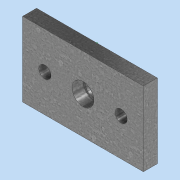
# Autodesk Inventor part: Unten
Saved by Autodesk Inventor 2021 (Build 250183000, 183)
## iProperties
Created: 2024-03-13
Part Number: Unten
Material: Generic
Document SubType Name: Modeling
Designer: Nokia
Density: 1 g/cm^3
Appearance: Steel Galvanized
Mass: 1145.79 g
Surface Area: 1212.7 cm^2
Volume: 1145.79 cm^3
Author: Nokia
Autodesk Inventor part; units mm, degrees
ref_plane "YZ Plane" through (0, 0, 0) normal (1, 0, 0) x (0, 1, 0)
ref_plane "XZ Plane" through (0, 0, 0) normal (0, 1, 0) x (-1, 0, 0)
ref_plane "XY Plane" through (0, 0, 0) normal (0, 0, 1) x (1, 0, 0)
sketch "Sketch1" plane through (0, 0, 0) normal (0, 0, 1) x (1, 0, 0)
  line L0 (130, -80) -> (130, 80)
  line L1 (130, 80) -> (-130, 80)
  line L2 (-130, 80) -> (-130, -80)
  line L3 (-130, -80) -> (130, -80)
  point P0 (0, 0)
  point P1 (0, 0)
  dimension "d0" = 260
  dimension "d1" = 160
  constraints: 8 end point, 3 perpendicular
  measures "d0" distance of L0.end L1.end
  measures "d1" distance of L1.end L2.end
extrude "Extrusion1" add sketch "Sketch1" along normal blind 30
sketch "Sketch2" plane through (0, 0, 30) normal (0, 0, 1) x (1, 0, 0)
  circle A0 centre (0, 0) radius 20
  circle A1 centre (0, 0) radius 23.5
  dimension "d4" = 40
  dimension "d5" = 47
  constraints: 2 centre point, 2 coincident
  measures "d4" diameter of A0
  measures "d5" diameter of A1
extrude "Extrusion2" cut sketch "Sketch2" against normal blind 30 contours A0
extrude "Extrusion3" cut sketch "Sketch2" against normal blind 24
sketch "Sketch3" plane through (0, 0, 30) normal (0, 0, 1) x (1, 0, 0)
  line L0 (-130, 80) -> (-130, -80) projected
  circle A0 centre (-82, 0) radius 13
  circle A1 centre (82, 0) radius 13
  line L1 (130, -80) -> (130, 80) projected
  point P0 (0, 0)
  dimension "d11" = 26
  dimension "d14" = 48
  dimension "d15" = 48
  constraints: 2 centre point
  measures "d11" diameter of A0
  measures "d14" distance from line of L0 A0.centre
  measures "d15" distance from line of L1 A1.centre
extrude "Extrusion4" cut sketch "Sketch3" against normal through all
sketch "Sketch4" plane through (-130, 80, 0) normal (0, 1, 0) x (1, 0, 0)
  point P0 (130, 0)
sketch "Sketch7" plane through (-130, -80, 0) normal (0, -1, 0) x (1, 0, 0)
  line L0 (260, 0) -> (0, 0)
  line L1 (0, 0) -> (0, 30)
  line L2 (130, 30) -> (260, 30)
  line L3 (130, 30) -> (130, 0)
  line L4 (195, 81.0719) -> (195, -34.56)
  line L5 (130, 15) -> (195, 15)
  line L6 (162.5, 115.0039) -> (162.5, -41.4165)
  circle A0 centre (162.5, 15) radius 14
  circle A1 centre (227.5, 15) radius 14
  circle A2 centre (32.5, 15) radius 14
  circle A3 centre (97.5, 15) radius 14
  circle A4 centre (162.5, 15) radius 7
  circle A5 centre (227.5, 15) radius 7
  circle A6 centre (32.5, 15) radius 7
  circle A7 centre (97.5, 15) radius 7
  line L7 (260, 0) -> (0, 0) projected
  point P0 (-260, 0)
  dimension "d16" = 30
  dimension "d17" = 28
  dimension "d18" = 14
  dimension "d19" = 0
  dimension "d21" = 0
  constraints: 14 end point, 8 centre point, 6 symmetric about line, 3 midpoint, 2 coincident, 2 perpendicular, 2 point on line, 1 parallel, 1 vertical, 7 other
  measures "d16" distance of L1.start L1.end
  measures "d17" diameter of A0
  measures "d18" diameter of A4
  measures "d19" distance of point (0, 0) L1.start
  measures "d21" distance from line of L1 point (0, 0)
hole "Hole1" at (97.5, -80, 15) at (32.5, -80, 15) at (-32.5, -80, 15) at (-97.5, -80, 15) direction (0, 1, 0) diameter 10.106 depth 65 tip angle 118 thread size "M12x1.75" class "6H" standard "ISO Metric profile"
body "Solid1"
